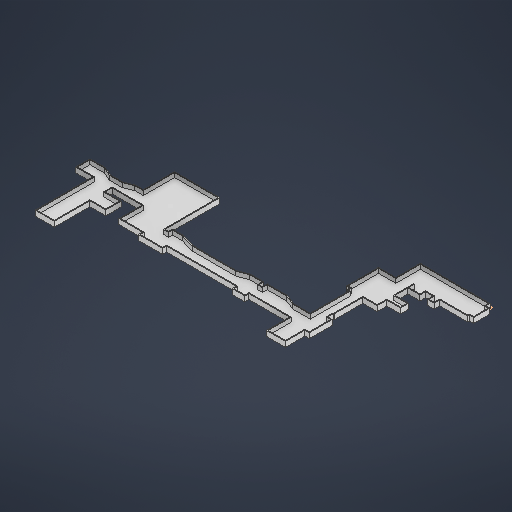
# Autodesk Inventor part: piso3
Saved by Autodesk Inventor 2026.1 (Build 301233020, 233B)
## iProperties
Created: 2025-10-08
Part Number: piso3
Material: Generic
Document SubType Name: Modeling
Designer: eduar
Density: 1 g/cm^3
Appearance: Default
Author: eduar
Autodesk Inventor part; units mm, degrees
ref_plane "YZ Plane" through (0, 0, 0) normal (1, 0, 0) x (0, 1, 0)
ref_plane "XZ Plane" through (0, 0, 0) normal (0, 1, 0) x (-1, 0, 0)
ref_plane "XY Plane" through (0, 0, 0) normal (0, 0, 1) x (1, 0, 0)
sketch "Sketch1" plane through (0, 0, 0) normal (0, 1, 0) x (-1, 0, 0)
  line L0 (0, 0) -> (15843, 0)
  line L1 (0, 972.6231) -> (0, 0)
  line L2 (0, 972.6231) -> (-908.158, 972.6231)
  line L3 (-908.158, 972.6231) -> (-908.158, 4329.8007)
  line L4 (0, 4329.8007) -> (-908.158, 4329.8007)
  line L5 (0, 4329.8007) -> (0, 4745.5862)
  line L6 (0, 4745.5862) -> (6580.8469, 4745.5862)
  line L7 (6580.8469, 6046.9734) -> (6580.8469, 4745.5862)
  line L8 (7754.4471, 6046.9734) -> (6580.8469, 6046.9734)
  line L9 (7754.4471, 6046.9734) -> (7754.4471, 4745.5862)
  line L10 (7754.4471, 4745.5862) -> (9897.7799, 4745.5862)
  line L11 (9897.7799, 6046.9734) -> (9897.7799, 4745.5862)
  line L12 (12501.7762, 6046.9734) -> (9897.7799, 6046.9734)
  line L13 (12501.7762, 6046.9734) -> (12501.7762, 4745.5862)
  line L14 (12708.8748, 4745.5862) -> (12501.7762, 4745.5862)
  line L15 (12708.8748, 4745.5862) -> (12708.8748, 9428.5348)
  line L16 (12708.8748, 9428.5348) -> (9529.2374, 9428.5348)
  line L17 (9529.2374, 10947.8541) -> (9529.2374, 9428.5348)
  line L18 (9529.2374, 10947.8541) -> (12708.8748, 10947.8541)
  line L19 (12708.8748, 13193.2861) -> (12708.8748, 10947.8541)
  line L20 (12708.8748, 13193.2861) -> (16066.5025, 13193.2861)
  line L21 (16066.5025, 13193.2861) -> (16066.5025, 19932.3451)
  line L22 (16066.5025, 19932.3451) -> (16196.818, 20035.8469)
  line L23 (16196.818, 21602.8668) -> (16196.818, 20035.8469)
  line L24 (15165.5521, 21602.8668) -> (16196.818, 21602.8668)
  line L25 (15165.5521, 21602.8668) -> (15165.5521, 26544.5184)
  line L26 (16196.818, 26544.5184) -> (15165.5521, 26544.5184)
  line L27 (16196.818, 31091.6041) -> (16196.818, 26544.5184)
  line L28 (20211.9494, 31091.6041) -> (16196.818, 31091.6041)
  line L29 (20211.9494, 25702.1028) -> (20211.9494, 31091.6041)
  line L30 (30097.7203, 25702.1028) -> (20211.9494, 25702.1028)
  line L31 (30097.7203, 25702.1028) -> (30097.7203, 26633.399)
  line L32 (32644.9685, 26633.399) -> (30097.7203, 26633.399)
  line L33 (32644.9685, 25702.1028) -> (32644.9685, 26633.399)
  line L34 (49310.1312, 25702.1028) -> (32644.9685, 25702.1028)
  line L35 (49310.1312, 26633.399) -> (49310.1312, 25702.1028)
  line L36 (54526.4608, 26633.399) -> (49310.1312, 26633.399)
  line L37 (54526.4608, 25702.1028) -> (54526.4608, 26633.399)
  line L38 (54526.4608, 25702.1028) -> (59992.2751, 25702.1028)
  line L39 (59992.2751, 20326.3088) -> (59992.2751, 25702.1028)
  line L40 (59992.2751, 20326.3088) -> (67368.4306, 20326.3088)
  line L41 (67368.4306, 20326.3088) -> (67368.4306, 22313.5879)
  line L42 (67368.4306, 22313.5879) -> (63655.5164, 22313.5879)
  line L43 (63655.5164, 25485.204) -> (63655.5164, 22313.5879)
  line L44 (67368.4306, 25485.204) -> (63655.5164, 25485.204)
  line L45 (67368.4306, 25485.204) -> (67368.4306, 33770.3623)
  line L46 (71450.3714, 33770.3623) -> (67368.4306, 33770.3623)
  line L47 (71450.3714, 20326.3088) -> (71450.3714, 33770.3623)
  line L48 (71450.3714, 20326.3088) -> (75432.8734, 20326.3088)
  line L49 (75432.8734, 17402.2155) -> (75432.8734, 20326.3088)
  line L50 (72086.4023, 17402.2155) -> (75432.8734, 17402.2155)
  line L51 (72086.4023, 17402.2155) -> (70059.1736, 18263.3147)
  line L52 (70059.1736, 18263.3147) -> (67099.7304, 18263.3147)
  line L53 (67099.7304, 18263.3147) -> (64990.7669, 17402.2155)
  line L54 (62988.8924, 17402.2155) -> (64990.7669, 17402.2155)
  line L55 (62988.8924, 10141.4101) -> (62988.8924, 17402.2155)
  line L56 (52836.678, 10141.4101) -> (62988.8924, 10141.4101)
  line L57 (52836.678, 22907.8802) -> (52836.678, 10141.4101)
  line L58 (51619.4586, 22907.8802) -> (52836.678, 22907.8802)
  line L59 (51619.4586, 21993.5806) -> (51619.4586, 22907.8802)
  line L60 (51619.4586, 21993.5806) -> (49299.602, 21993.5806)
  line L61 (49299.602, 21993.5806) -> (46152.8439, 22907.8802)
  line L62 (46152.8439, 22907.8802) -> (41732.2616, 22907.8802)
  line L63 (41732.2616, 22907.8802) -> (36009.3179, 22907.8802)
  line L64 (36009.3179, 22907.8802) -> (33581.57, 21993.5806)
  line L65 (30719.5233, 21993.5806) -> (33581.57, 21993.5806)
  line L66 (30719.5233, 23101.1734) -> (30719.5233, 21993.5806)
  line L67 (29577.3124, 23101.1734) -> (30719.5233, 23101.1734)
  line L68 (29577.3124, 21993.5806) -> (29577.3124, 23101.1734)
  line L69 (29577.3124, 21993.5806) -> (25036.7234, 21993.5806)
  line L70 (22662.4162, 22907.8802) -> (25036.7234, 21993.5806)
  line L71 (18594.647, 22907.8802) -> (22662.4162, 22907.8802)
  line L72 (18594.647, 22907.8802) -> (18594.647, 13596.3685)
  line L73 (19033.7894, 13596.3685) -> (18594.647, 13596.3685)
  line L74 (19033.7894, 12786.5405) -> (19033.7894, 13596.3685)
  line L75 (19889.5196, 12786.5405) -> (19033.7894, 12786.5405)
  line L76 (19889.5196, 5707.1291) -> (19889.5196, 12786.5405)
  line L77 (19889.5196, 5707.1291) -> (15843, 5707.1291)
  line L78 (15843, 0) -> (15843, 5707.1291)
  dimension "d0" = 15843
  dimension "d1" = 5707.1291
  constraints: 158 end point, 69 perpendicular, 16 collinear, 2 horizontal, 1 vertical
  measures "d0" distance of L0.start L0.end
  measures "d1" distance of L0.end L77.end
extrude "Extrusion1" add sketch "Sketch1" along normal blind 1000
shell "Shell1" thickness 200 outward yes removed faces 1 at (-55221.877, 1000, 17791.8664)
body "Solid1"
